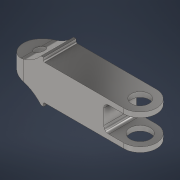
# Autodesk Inventor part: holder3_l4
Saved by Autodesk Inventor 2021 (Build 250183000, 183)
## iProperties
Created: 2021-06-13
Part Number: holder3_l4
Material: Steel, High Strength, Low Alloy
Document SubType Name: Modeling
Designer: Watchdog
Density: 7.85 g/cm^3
Appearance: Steel - Polished
Mass: 50.8737 g
Surface Area: 29.4737 cm^2
Volume: 6.48072 cm^3
Author: Watchdog
Autodesk Inventor part; units mm, degrees
ref_plane "YZ Plane" through (0, 0, 0) normal (1, 0, 0) x (0, 1, 0)
ref_plane "XZ Plane" through (0, 0, 0) normal (0, 1, 0) x (-1, 0, 0)
ref_plane "XY Plane" through (0, 0, 0) normal (0, 0, 1) x (1, 0, 0)
sketch "Sketch1" plane through (0, 0, 0) normal (0, 1, 0) x (-1, 0, 0)
  line L0 (20, -6.5) -> (-20, -6.5)
  line L1 (-20, 6.5) -> (20, 6.5)
  arc A0 (20, -6.5) -> (20, 6.5) centre (20, 0) ccw
  arc A1 (-20, 6.5) -> (-20, -6.5) centre (-20, 0) ccw
  point P0 (0, 0)
  dimension "d0" = 13
  dimension "d2" = 6.5
  dimension "d4" = 40
  dimension "d5" = 20
  constraints: 4 end point, 4 point on circle, 4 tangent, 2 centre point, 1 horizontal
  measures "d0" distance between parallel lines of L1 L0
  measures "d2" distance from line of point (0, 0) L0
  measures "d4" distance of L0.end L0.start
  measures "d5" horizontal distance of point (0, 0) L0.start
extrude "Extrusion1" add sketch "Sketch1" along normal mid plane 14
sketch "Sketch2" plane through (0, 7, 0) normal (0, 1, 0) x (1, 0, 0)
  arc A0 (-20, 6.5) -> (-20, -6.5) centre (-20, 0) ccw projected
  arc A1 (20, -6.5) -> (20, 6.5) centre (20, 0) ccw projected
  point P0 (0, 0)
  point P1 (20, 0)
  dimension "d9" = 0
  dimension "d12" = 0
  measures "d9" vertical distance of point (0, 0) point (20, 0)
  measures "d12" distance of A1.centre point (20, 0)
ref_plane "midPlane" through (-20, -7, 0) normal (0, 0, 1) x (1, 0, 0)
sketch "Sketch5" plane through (-20, 7, 6.5) normal (0, 0, 1) x (1, 0, 0)
  line L0 (32, -2) -> (60, -2)
  line L1 (60, -2) -> (60, -12)
  line L2 (60, -12) -> (32, -12)
  line L3 (32, -12) -> (32, -2)
  line L4 (40, -14) -> (0, -14) projected
  line L5 (0, 0) -> (40, 0) projected
  line L6 (46.5, 0) -> (40, 0) projected
  line L7 (40, -14) -> (40, 0) projected
  dimension "d35" = 14
  dimension "d36" = 10
  dimension "d37" = 2
  dimension "d38" = 8
  dimension "d39" = 20
  constraints: 8 end point, 2 parallel, 1 horizontal, 1 perpendicular
  measures "d35" distance between parallel lines of L4 L5
  measures "d36" distance of L2.end L0.start
  measures "d37" distance between parallel lines of L6 L0
  measures "d38" distance between parallel lines of L7 L3
  measures "d39" distance between parallel lines of L7 L1
extrude "Extrusion4" cut sketch "Sketch5" against normal through all
hole "Hole2" at (20, 7, 0) direction (0, -1, 0) diameter 5 depth 2 counterbore diameter 7 counterbore depth 2
sketch "Sketch8" plane through (0, 7, 0) normal (0, 1, 0) x (1, 0, 0)
  arc A0 (-20, 6.5) -> (-20, -6.5) centre (-20, 0) ccw projected
  point P0 (0, 0)
  constraints: 1 coincident
sketch "Sketch9" plane through (0, -7, 0) normal (0, -1, 0) x (1, 0, 0)
  arc A0 (20, -6.5) -> (20, 6.5) centre (20, 0) ccw projected
  point P0 (0, 0)
  constraints: 1 coincident
hole "Hole3" at (20, -7, 0) direction (0, 1, 0) diameter 6 depth 2 counterbore diameter 8 counterbore depth 2
hole "Hole4" at (-20, 7, 0) direction (0, -1, 0) diameter 4 end through all
fillet "Fillet3" radius 2 2 edges at (12, 5, 0) (12, -5, 0)
sketch "Sketch10" plane through (0, 7, 0) normal (0, 1, 0) x (1, 0, 0)
  line L0 (-20, 6.5) -> (20, 6.5) projected
  line L1 (20, -6.5) -> (-20, -6.5) projected
  line L2 (-13, 6.5) -> (-12, 6.5)
  line L3 (-12, 6.5) -> (-12, -6.5)
  line L4 (-12, -6.5) -> (-13, -6.5)
  line L5 (-13, -6.5) -> (-13, 6.5)
  circle A0 centre (-20, 0) radius 2 projected
  point P0 (0, 0)
  dimension "d70" = 7
  dimension "d71" = 1
  constraints: 8 end point, 2 parallel, 2 point on line, 1 horizontal, 1 perpendicular
  measures "d70" distance from line of A0.centre L5
  measures "d71" distance between parallel lines of L5 L3
extrude "Extrusion7" add sketch "Sketch10" along normal blind 1.5 contours L0 L3 L1 L5
sketch "Sketch11" plane through (0, -7, 0) normal (0, -1, 0) x (1, 0, 0)
  line L0 (-13, 6.5) -> (-12, 6.5) projected
  line L1 (-12, 6.5) -> (-12, -6.5) projected
  line L2 (-12, -6.5) -> (-13, -6.5) projected
  line L3 (-13, -6.5) -> (-13, 6.5) projected
  point P0 (0, 0)
extrude "Extrusion8" add sketch "Sketch11" along normal blind 1.5
sketch "Sketch12" plane through (-20, -7, -6.5) normal (0, 0, -1) x (-1, 0, 0)
  line L0 (6.5, 0) -> (6.5, 14) projected
  line L1 (0, 0) -> (-7, 0) projected
  arc A0 (6.5, 4) -> (-7, 0) centre (6.5648, -20.9999) ccw
  line L2 (6.5, 14) -> (0, 14) projected
  line L3 (0, 0) -> (6.5, 0) projected
  line L4 (-7, 14) -> (-7, 15.5) projected
  arc A1 (-7, 14) -> (6.5, 10) centre (6.5648, 34.9999) ccw
  point P0 (-20, 7)
  dimension "d78" = 25
  dimension "d79" = 14
  dimension "d80" = 25
  dimension "d81" = 6
  dimension "d82" = 4
  constraints: 4 point on circle, 2 centre point, 2 point on line
  measures "d78" radius of A0
  measures "d79" distance between parallel lines of L2 L3
  measures "d80" radius of A1
  measures "d81" distance of A0.start A1.end
  measures "d82" distance from line of L3 A0.start
extrude "Extrusion9" cut sketch "Sketch12" against normal through all
ref_plane "lateralPlane" through (0, 0, 0) normal (0, -1, 0) x (1, 0, 0)
fillet "Fillet6" radius 15 1 edges at (-13, -7, 0)
mirror "Mirror1" about plane through (0, 0, 0) normal (0, -1, 0) of "Fillet6", "Extrusion9"
fillet "Fillet7" radius 0.5 2 edges at (-12, -7, 0) (-12, 7, 0)
equation "\"d2\" = 0.5 * d0"
equation "\"d5\" = 0.5 * d4"
equation "\"d37\" = -0.5 * d36 + 0.5 * d35"
equation "\"d80\" = d78"
equation "\"d82\" = -0.5 * d81 + 0.5 * d79"
body "Solid1"
